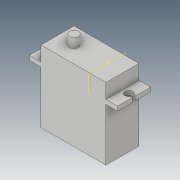
# Autodesk Inventor part: gripperServo
Saved by Autodesk Inventor 2018 (Build 220112000, 112)
## iProperties
Created: 2020-01-19
Part Number: gripperServo
Material: Generic
Document SubType Name: Modeling
Designer: anirudh
Density: 1 g/cm^3
Appearance: Default
Author: anirudh
Autodesk Inventor part; units mm, degrees
ref_plane "YZ Plane" through (0, 0, 0) normal (1, 0, 0) x (0, 1, 0)
ref_plane "XZ Plane" through (0, 0, 0) normal (0, 1, 0) x (-1, 0, 0)
ref_plane "XY Plane" through (0, 0, 0) normal (0, 0, 1) x (1, 0, 0)
sketch "Sketch1" plane through (0, 0, 0) normal (0, 1, 0) x (-1, 0, 0)
  line L0 (0, 0) -> (-29.5, 0)
  line L1 (-29.5, 0) -> (-29.5, -15)
  line L2 (-29.5, -15) -> (0, -15)
  line L3 (0, -15) -> (0, 0)
  dimension "d2" = 29.5
  dimension "d3" = 15
  constraints: 8 end point, 2 parallel, 1 horizontal, 1 perpendicular
  measures "d2" distance of L2.end L1.end
  measures "d3" distance of L1.end L0.end
extrude "Extrusion1" add sketch "Sketch1" along normal blind 23.85
ref_plane "Work Plane1" through (0, 23.85, 0) normal (0, 1, 0) x (1, 0, 0)
sketch "Sketch2" plane through (0, 23.85, 0) normal (0, 1, 0) x (1, 0, 0)
  line L0 (0, 0) -> (29.5, 0) projected
  line L1 (0, 0) -> (-5.25, 0)
  line L2 (29.5, 15) -> (0, 15) projected
  line L3 (-5.25, 15) -> (29.5, 15)
  line L4 (29.5, 15) -> (34.75, 15)
  line L5 (34.75, 0) -> (0, 0)
  arc A0 (-4.4155, 6.625) -> (-4.4155, 8.375) centre (-2.9, 7.5) ccw
  arc A1 (33.9155, 8.375) -> (33.9155, 6.625) centre (32.4, 7.5) ccw
  line L6 (-4.4155, 6.625) -> (-5.25, 6.625)
  line L7 (-4.4155, 8.375) -> (-5.25, 8.375)
  line L8 (33.9155, 6.625) -> (34.75, 6.625)
  line L9 (33.9155, 8.375) -> (34.75, 8.375)
  line L10 (34.75, 15) -> (34.75, 8.375)
  line L11 (34.75, 6.625) -> (34.75, 0)
  line L12 (-5.25, 0) -> (-5.25, 6.625)
  line L13 (-5.25, 8.375) -> (-5.25, 15)
  dimension "d7" = 5.25
  dimension "d8" = 5.25
  dimension "d14" = 3.5
  dimension "d15" = 3.5
  constraints: 24 end point, 8 perpendicular, 4 point on circle, 4 point on line, 2 centre point, 1 collinear, 1 horizontal
  measures "d7" distance of L0.start L1.end
  measures "d8" distance of L2.start L4.end
  measures "d14" diameter of A0
  measures "d15" diameter of A1
extrude "Extrusion2" add sketch "Sketch2" along normal blind 2
sketch "Sketch3" plane through (0, 23.85, 0) normal (0, 1, 0) x (1, 0, 0)
  line L0 (0, 0) -> (29.5, 0) projected
  line L1 (29.5, 0) -> (29.5, 15) projected
  line L2 (0, 0) -> (29.5, 0)
  line L3 (29.5, 0) -> (29.5, 15)
  line L4 (29.5, 15) -> (0, 15)
  line L5 (0, 15) -> (0, 0)
  constraints: 8 end point, 2 parallel, 1 horizontal, 1 perpendicular
extrude "Extrusion3" add sketch "Sketch3" along normal blind 8.65
sketch "Sketch4" plane through (0, 32.5, 0) normal (0, 1, 0) x (1, 0, 0)
  circle A0 centre (7.5, 7.5) radius 2
  point P0 (0, 0)
  dimension "d22" = 4
  constraints: 1 centre point
  measures "d22" diameter of A0
extrude "Extrusion4" add sketch "Sketch4" along normal blind 4.35
sketch "Sketch6" plane through (0, 32.5, 0) normal (0, 1, 0) x (1, 0, 0)
  circle A0 centre (7.5, 7.5) radius 2 projected
  circle A1 centre (7.5, 7.5) radius 14.989
  line L0 (7.5, 7.5) -> (22.489, 7.5)
  point P0 (0, 0)
  dimension "d28" = 29.978
  constraints: 2 end point, 1 coincident, 1 horizontal, 1 horizontal alignment, 2 other
ref_plane "Work Plane3" through (22.4896, 25.85, -15) normal (1, 0, 0) x (0, 0, -1)
body "Solid1"
